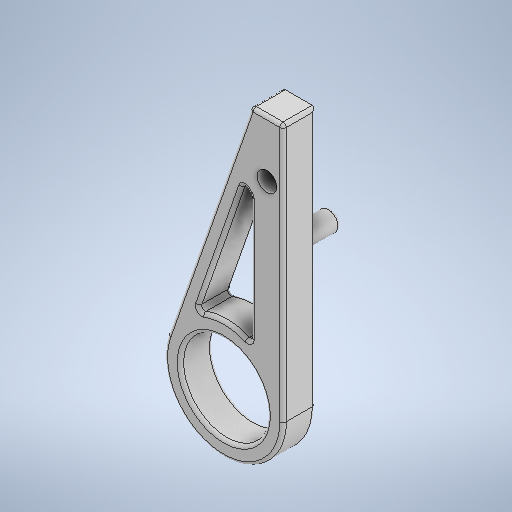
# Autodesk Inventor part: Pedal Support R
Saved by Autodesk Inventor 2025.2 (Build 292293000, 293)
## iProperties
Created: 2025-03-16
Part Number: Pedal Support R
Material: Generic
Document SubType Name: Modeling
Designer: eason
Density: 1 g/cm^3
Appearance: Default
Author: eason
Autodesk Inventor part; units mm, degrees
ref_plane "YZ Plane" through (0, 0, 0) normal (1, 0, 0) x (0, 1, 0)
ref_plane "XZ Plane" through (0, 0, 0) normal (0, 1, 0) x (-1, 0, 0)
ref_plane "XY Plane" through (0, 0, 0) normal (0, 0, 1) x (1, 0, 0)
sketch "Sketch1" plane through (0, 0, 0) normal (0, 0, 1) x (1, 0, 0)
  circle A0 centre (-18.4, 0) radius 13.4
  arc A1 (-35.7747, 6.0563) -> (0, 0) centre (-18.4, 0) ccw
  line L0 (-35.7747, 6.0563) -> (-10, 80)
  line L1 (0, 0) -> (0, 80)
  line L2 (0, 80) -> (-10, 80)
  line L3 (0, -41.4558) -> (0, 100.2426) projected
  line L4 (-47.5867, 0) -> (8.228, 0) projected
  dimension "d0" = 26.8
  dimension "d1" = 5
  dimension "d2" = 80
  dimension "d8" = 10
  constraints: 6 end point, 2 centre point, 2 point on circle, 2 tangent, 1 coincident, 1 collinear, 1 perpendicular, 1 point on line
  measures "d0" diameter of A0
  measures "d1" radial gap between concentric circles of A1 A0
  measures "d2" distance from line of L1.start L2
  measures "d8" distance of L2.start L0.end
extrude "Extrusion1" add sketch "Sketch1" along normal blind 10 contours L4 A1 A0 | A0 L4 A1 L0 L2 L1
sketch "Sketch4" plane through (0, 0, 10) normal (0, 0, 1) x (1, 0, 0)
  circle A0 centre (-5, 62.5) radius 3
  circle A1 centre (-5, 42.5) radius 3
  line L0 (-5, 42.5) -> (-5, 80) construction
  line L1 (0, 80) -> (-10, 80) projected
  line L2 (0, 0) -> (0, 80) projected
  dimension "d23" = 6
  dimension "d24" = 6
  dimension "d25" = 17.5
  dimension "d26" = 20
  constraints: 2 centre point, 2 end point, 1 midpoint, 1 parallel, 1 point on line
  measures "d23" diameter of A0
  measures "d24" diameter of A1
  measures "d25" distance from line of L1 A0.centre
  measures "d26" distance of L0.start A0.centre
extrude "Extrusion5" cut sketch "Sketch4" against normal up to surface (10 mm away) contours A0
sketch "Sketch5" plane through (0, 0, 0) normal (0, 0, -1) x (-1, 0, 0)
  circle A0 centre (5, 42.5) radius 3 projected
  point P0 (0, 0)
extrude "Extrusion7" add sketch "Sketch5" along normal blind 10
sketch "Sketch6" plane through (0, 0, 0) normal (0, 0, -1) x (-1, 0, 0)
  arc A0 (26.9029, 16.3175) -> (10, 16.3707) centre (18.4, 0) ccw
  line L0 (10, 36.255) -> (10, 16.3707)
  line L1 (0, 0) -> (0, 80) projected
  circle A1 centre (5, 42.5) radius 3 projected
  circle A2 centre (18.4, 0) radius 13.4 projected
  line L2 (10, 80) -> (35.7747, 6.0563) projected
  line L3 (0, 0) -> (0, 80) projected
  line L4 (10, 36.255) -> (10, 56.255)
  line L5 (26.9029, 16.3175) -> (8.2581, 69.8065)
  arc A3 (10, 56.255) -> (8.2581, 69.8065) centre (5, 62.5) ccw
  circle A4 centre (5, 62.5) radius 3 projected
  point P0 (12.094, 58.802)
  dimension "d36" = 5
  dimension "d40" = 10
  dimension "d43" = 5
  dimension "d44" = 5
  constraints: 6 end point, 4 point on circle, 2 centre point, 2 concentric, 2 parallel, 1 collinear, 1 vertical
  measures "d36" radial gap between concentric circles of A2 A0
  measures "d40" distance between parallel lines of L1 L0
  measures "d43" radial gap between concentric circles of A4 A3
  measures "d44" distance between parallel lines of L5 L2
extrude "Extrusion8" cut sketch "Sketch6" against normal up to surface (10 mm away) contours A0 L0 L4 A3 L5
fillet "Fillet1" radius 1 12 edges at (-21.4713, -18.1419, 10) (0, 40, 10) (-22.8874, 43.0282, 10) (-21.4713, -18.1419, 0) (0, 40, 0) (-22.8874, 43.0282, 0) (-2, 42.5, -10) (-31.8, 0, 10) (-31.8, 0, 0) (-10, 80, 5) (-5, 80, 10) (0, 80, 5)
fillet "Fillet2" radius 1 4 edges at (-12.094, 58.802, 5) (-10, 56.255, 5) (-10, 16.3707, 5) (-26.9029, 16.3175, 5)
fillet "Fillet3" radius 1 16 edges at (-10.4439, 17.1021, 10) (-18.0933, 18.3974, 10) (-25.8973, 17.4548, 10) (-19.4438, 37.7166, 10) (-11.989, 57.5872, 10) (-10.7007, 56.8873, 10) (-10.0871, 56.2, 10) (-10, 36.8625, 10) (-10.4439, 17.1021, 0) (-10, 36.8625, 0) (-10.0871, 56.2, 0) (-18.0933, 18.3974, 0) (-10.7007, 56.8873, 0) (-25.8973, 17.4548, 0) (-11.989, 57.5872, 0) (-19.4438, 37.7166, 0)
body "Solid1"
